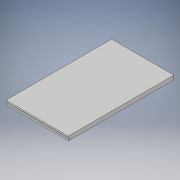
# Autodesk Inventor part: planche
Saved by Autodesk Inventor 2017 (Build 210142000, 142)
## iProperties
Created: 2018-11-15
Part Number: planche
Material: Generic
Document SubType Name: Modeling
Designer: Antoine Blaud
Density: 1 g/cm^3
Appearance: Default
Author: Antoine Blaud
Autodesk Inventor part; units mm, degrees
ref_plane "YZ Plane" through (0, 0, 0) normal (1, 0, 0) x (0, 1, 0)
ref_plane "XZ Plane" through (0, 0, 0) normal (0, 1, 0) x (-1, 0, 0)
ref_plane "XY Plane" through (0, 0, 0) normal (0, 0, 1) x (1, 0, 0)
sketch "Sketch1" plane through (0, 0, 0) normal (1, 0, 0) x (0, 1, 0)
  line L0 (0, 0) -> (-10.16, 0)
  line L1 (-10.16, 0) -> (-10.16, -254)
  line L2 (-10.16, -254) -> (0, -254)
  line L3 (0, -254) -> (0, 0)
  dimension "d0" = 254
  dimension "d1" = 10.16
  constraints: 8 end point, 2 parallel, 1 horizontal, 1 perpendicular
  measures "d0" distance of L0.end L1.end
  measures "d1" distance between parallel lines of L3 L1
extrude "Extrusion1" add sketch "Sketch1" along normal blind 150
sketch "Sketch2" plane through (150, 0, 0) normal (1, 0, 0) x (0, 0, -1)
  line L0 (0, -3.175) -> (2.54, -3.175)
  line L1 (2.54, -3.175) -> (2.54, -6.985)
  line L2 (2.54, -6.985) -> (0, -6.985)
  line L3 (0, -6.985) -> (0, -3.175)
  line L4 (0, -10.16) -> (254, -10.16) projected
  line L5 (254, 0) -> (0, 0) projected
  line L6 (254, -3.175) -> (251.9121, -3.175)
  line L7 (251.9121, -3.175) -> (251.9121, -6.985)
  line L8 (251.9121, -6.985) -> (254, -6.985)
  line L9 (254, -6.985) -> (254, -3.175)
  dimension "d4" = 10.16
  dimension "d5" = 3.175
  dimension "d6" = 3.81
  dimension "d7" = 2.54
  dimension "d8" = 3.175
  dimension "d9" = 3.81
  dimension "d10" = 2.0879
  dimension "d11" = 251.46
  dimension "d12" = 0
  constraints: 16 end point, 4 parallel, 2 horizontal, 2 perpendicular
  measures "d4" distance between parallel lines of L4 L5
  measures "d5" distance between parallel lines of L0 L5
  measures "d6" distance between parallel lines of L2 L0
  measures "d7" distance between parallel lines of L3 L1
  measures "d8" distance between parallel lines of L6 L5
  measures "d9" distance between parallel lines of L8 L6
  measures "d10" distance between parallel lines of L9 L7
  measures "d11" distance between parallel lines of L9 L1
  measures "d12" distance from line of L5.start L9
extrude "Extrusion2" cut sketch "Sketch2" against normal blind 150
body "Solid1"
